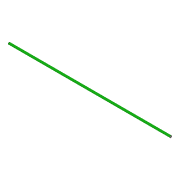
# Autodesk Inventor part: Carry_Pole
Saved by Autodesk Inventor 2019.3 (Build 233278000, 278)
## iProperties
Created: 2019-01-16
Part Number: Carry_Pole
Material: Steel, Galvanized
Document SubType Name: Modeling
Designer: Kathryn Rosie
Density: 7.85 g/cm^3
Appearance: Galvanized
Mass: 5326.88 g
Surface Area: 4529.32 cm^2
Volume: 678.584 cm^3
Author: Kathryn Rosie
Autodesk Inventor part; units mm, degrees
ref_plane "YZ Plane" through (0, 0, 0) normal (1, 0, 0) x (0, 1, 0)
ref_plane "XZ Plane" through (0, 0, 0) normal (0, 1, 0) x (-1, 0, 0)
ref_plane "XY Plane" through (0, 0, 0) normal (0, 0, 1) x (1, 0, 0)
sketch "Sketch1" plane through (0, 0, 0) normal (1, 0, 0) x (0, 1, 0)
  circle A0 centre (0, 0) radius 15.9
  circle A1 centre (0, 0) radius 12.9
  dimension "d0" = 31.8
  dimension "d1" = 3
  constraints: 2 centre point, 1 coincident
  measures "d0" diameter of A0
  measures "d1" radial gap between concentric circles of A0 A1
extrude "Extrusion1" add sketch "Sketch1" along normal blind 2500
body "Solid1"
